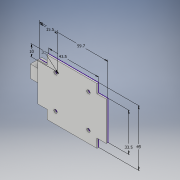
# Autodesk Inventor part: Protoboard
Saved by Autodesk Inventor 2019.3 (Build 233278000, 278)
## iProperties
Created: 2019-06-06
Part Number: Protoboard
Material: Generic
Document SubType Name: Modeling
Designer: Frienddo
Density: 1 g/cm^3
Appearance: Default
Author: Frienddo
Autodesk Inventor part; units mm, degrees
ref_plane "YZ Plane" through (0, 0, 0) normal (1, 0, 0) x (0, 1, 0)
ref_plane "XZ Plane" through (0, 0, 0) normal (0, 1, 0) x (-1, 0, 0)
ref_plane "XY Plane" through (0, 0, 0) normal (0, 0, 1) x (1, 0, 0)
sketch "Sketch1" plane through (0, 0, 0) normal (0, 0, 1) x (1, 0, 0)
  line L0 (0, 0) -> (-29.85, 0)
  line L1 (-29.85, 0) -> (-29.85, 16.75)
  line L2 (-29.85, 16.75) -> (-21.75, 16.75)
  line L3 (-21.75, 16.75) -> (-21.75, 24.5)
  line L4 (-21.75, 24.5) -> (0, 24.5)
  line L5 (0, 24.5) -> (0, 0)
  circle A0 centre (-14.35, 14.5) radius 1.5
  line L6 (0, 0) -> (29.85, 0)
  line L7 (29.85, 0) -> (29.85, 16.75)
  line L8 (29.85, 16.75) -> (21.75, 16.75)
  line L9 (21.75, 16.75) -> (21.75, 24.5)
  line L10 (21.75, 24.5) -> (0, 24.5)
  circle A1 centre (14.35, 14.5) radius 1.5
  line L11 (-29.85, 0) -> (-29.85, -16.75)
  line L12 (-29.85, -16.75) -> (-21.75, -16.75)
  line L13 (-21.75, -16.75) -> (-21.75, -24.5)
  line L14 (-21.75, -24.5) -> (0, -24.5)
  line L15 (0, -24.5) -> (0, 0)
  circle A2 centre (-14.35, -14.5) radius 1.5
  line L16 (29.85, 0) -> (29.85, -16.75)
  line L17 (29.85, -16.75) -> (21.75, -16.75)
  line L18 (21.75, -16.75) -> (21.75, -24.5)
  line L19 (21.75, -24.5) -> (0, -24.5)
  circle A3 centre (14.35, -14.5) radius 1.5
  dimension "d0" = 15.5
  dimension "d1" = 10
  dimension "d2" = 43.5
  dimension "d3" = 59.7
  dimension "d4" = 49
  dimension "d5" = 33.5
  dimension "d6" = 3
  constraints: 40 end point, 14 symmetric about line, 5 perpendicular, 4 centre point, 1 horizontal, 3 other
  measures "d0" distance from line of L1 A0.centre
  measures "d1" distance from line of L4 A0.centre
  measures "d2" distance between parallel lines of L3 L9
  measures "d3" distance between parallel lines of L7 L1
  measures "d4" distance between parallel lines of L19 L10
  measures "d5" distance between parallel lines of L17 L8
  measures "d6" diameter of A0
ref_plane "Work Plane1" through (0, 0, 0) normal (0, 0, -1) x (-1, 0, 0)
extrude "Extrusion1" add sketch "Sketch1" along normal blind 1.5
sketch "Sketch3" plane through (0, 0, 0) normal (0, 0, 1) x (1, 0, 0)
  line L0 (-21.85, 8.75) -> (-37.85, 8.75)
  line L1 (-37.85, 8.75) -> (-37.85, -2.25)
  line L2 (-37.85, -2.25) -> (-21.85, -2.25)
  line L3 (-21.85, -2.25) -> (-21.85, 8.75)
  line L4 (-21.75, 16.75) -> (-29.85, 16.75) projected
  line L5 (-29.85, 16.75) -> (-29.85, -16.75) projected
  point P0 (0, 0)
  dimension "d19" = 8
  dimension "d20" = 11
  dimension "d21" = 8
  constraints: 8 end point, 2 parallel, 1 horizontal, 1 perpendicular, 1 other
  measures "d19" distance between parallel lines of L4 L0
  measures "d20" distance of L0.end L1.end
  measures "d21" distance between parallel lines of L5 L3
extrude "Extrusion5" add sketch "Sketch3" against normal blind 10
body "Solid1"
